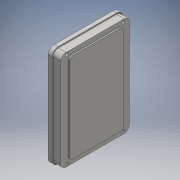
# Autodesk Inventor part: ET6
Saved by Autodesk Inventor 2016 (Build 200138000, 138)
## iProperties
Created: 2016-03-20
Part Number: ET6
Material: Genérico
Document SubType Name: Modeling
Designer: Usuario1
Density: 1 g/cm^3
Appearance: Valor por defecto
Author: Usuario1
Autodesk Inventor part; units mm, degrees
ref_plane "YZ Plane" through (0, 0, 0) normal (1, 0, 0) x (0, 1, 0)
ref_plane "XZ Plane" through (0, 0, 0) normal (0, 1, 0) x (-1, 0, 0)
ref_plane "XY Plane" through (0, 0, 0) normal (0, 0, 1) x (1, 0, 0)
sketch "Boceto1" plane through (0, 0, 0) normal (1, 0, 0) x (0, 1, 0)
  circle A0 centre (0.2799, 0.1054) radius 0.0623
  circle A1 centre (2.483, 0.1054) radius 0.0623
  circle A2 centre (2.483, -3.5918) radius 0.0623
  line L0 (0.3357, -3.3718) -> (0.3357, -0.1146)
  arc A3 (0.3357, -3.3718) -> (0.4557, -3.4918) centre (0.4557, -3.3718) ccw
  line L1 (0.4557, 0.0054) -> (2.3072, 0.0054)
  arc A4 (0.4557, 0.0054) -> (0.3357, -0.1146) centre (0.4557, -0.1146) ccw
  arc A5 (2.4272, -0.1146) -> (2.3072, 0.0054) centre (2.3072, -0.1146) ccw
  line L2 (2.4272, -0.1146) -> (2.4272, -3.3718)
  arc A6 (2.3072, -3.4918) -> (2.4272, -3.3718) centre (2.3072, -3.3718) ccw
  line L3 (2.3072, -3.4918) -> (0.4557, -3.4918)
  line L4 (0, -3.4863) -> (0, 0)
  arc A7 (0.24, 0.24) -> (0, 0) centre (0.24, 0) ccw
  line L5 (0.24, 0.24) -> (2.5229, 0.24)
  arc A8 (2.7629, 0) -> (2.5229, 0.24) centre (2.5229, 0) ccw
  line L6 (2.7629, 0) -> (2.7629, -3.4863)
  arc A9 (2.5229, -3.7263) -> (2.7629, -3.4863) centre (2.5229, -3.4863) ccw
  line L7 (2.5229, -3.7263) -> (0.24, -3.7263)
  arc A10 (0, -3.4863) -> (0.24, -3.7263) centre (0.24, -3.4863) ccw
  line L8 (2.7186, -3.4821) -> (2.7186, -0.0043)
  arc A11 (2.7186, -0.0043) -> (2.5186, 0.1957) centre (2.5186, -0.0043) ccw
  line L9 (2.5186, 0.1957) -> (0.2443, 0.1957)
  arc A12 (0.2443, 0.1957) -> (0.0443, -0.0043) centre (0.2443, -0.0043) ccw
  line L10 (0.0443, -0.0043) -> (0.0443, -3.4821)
  arc A13 (0.0443, -3.4821) -> (0.2443, -3.6821) centre (0.2443, -3.4821) ccw
  line L11 (0.2443, -3.6821) -> (2.5186, -3.6821)
  arc A14 (2.5186, -3.6821) -> (2.7186, -3.4821) centre (2.5186, -3.4821) ccw
  circle A15 centre (0.2799, -3.5918) radius 0.0623
  constraints: 24 end point, 24 point on circle, 16 centre point
extrude "Extrusión1" add sketch "Boceto1" along normal blind 0.15 contours L0 A4 L1 A5 L2 A6 L3 A3 | L4 A7 L5 A8 L6 A9 L7 A10 | A14 L11 A13 L10 A12 L9 A11 L8
sketch "Boceto2" plane through (0.15, 0, 0) normal (1, 0, 0) x (0, 0, -1)
  circle A0 centre (3.5918, 2.483) radius 0.0623
  circle A1 centre (3.5918, 0.2799) radius 0.0623
  circle A2 centre (-0.1054, 0.2799) radius 0.0623
  line L0 (0.1146, 2.4272) -> (3.3718, 2.4272)
  arc A3 (0.1146, 2.4272) -> (-0.0054, 2.3072) centre (0.1146, 2.3072) ccw
  line L1 (3.4918, 2.3072) -> (3.4918, 0.4557)
  arc A4 (3.4918, 2.3072) -> (3.3718, 2.4272) centre (3.3718, 2.3072) ccw
  arc A5 (3.3718, 0.3357) -> (3.4918, 0.4557) centre (3.3718, 0.4557) ccw
  line L2 (3.3718, 0.3357) -> (0.1146, 0.3357)
  arc A6 (-0.0054, 0.4557) -> (0.1146, 0.3357) centre (0.1146, 0.4557) ccw
  line L3 (-0.0054, 0.4557) -> (-0.0054, 2.3072)
  line L4 (0, 2.7629) -> (3.4863, 2.7629)
  arc A7 (3.7263, 2.5229) -> (3.4863, 2.7629) centre (3.4863, 2.5229) ccw
  line L5 (3.7263, 2.5229) -> (3.7263, 0.24)
  arc A8 (3.4863, 0) -> (3.7263, 0.24) centre (3.4863, 0.24) ccw
  line L6 (3.4863, 0) -> (0, 0)
  arc A9 (-0.24, 0.24) -> (0, 0) centre (0, 0.24) ccw
  line L7 (-0.24, 0.24) -> (-0.24, 2.5229)
  arc A10 (0, 2.7629) -> (-0.24, 2.5229) centre (0, 2.5229) ccw
  line L8 (0.0043, 0.0443) -> (3.4821, 0.0443)
  arc A11 (3.4821, 0.0443) -> (3.6821, 0.2443) centre (3.4821, 0.2443) ccw
  line L9 (3.6821, 0.2443) -> (3.6821, 2.5186)
  arc A12 (3.6821, 2.5186) -> (3.4821, 2.7186) centre (3.4821, 2.5186) ccw
  line L10 (3.4821, 2.7186) -> (0.0043, 2.7186)
  arc A13 (0.0043, 2.7186) -> (-0.1957, 2.5186) centre (0.0043, 2.5186) ccw
  line L11 (-0.1957, 2.5186) -> (-0.1957, 0.2443)
  arc A14 (-0.1957, 0.2443) -> (0.0043, 0.0443) centre (0.0043, 0.2443) ccw
  circle A15 centre (-0.1054, 2.483) radius 0.0623
  circle A16 centre (3.5918, 0.2799) radius 0.0623 projected
  circle A17 centre (3.5918, 2.483) radius 0.0623 projected
  circle A18 centre (-0.1054, 2.483) radius 0.0623 projected
  circle A19 centre (-0.1054, 0.2799) radius 0.0623 projected
  line L12 (0, 0) -> (3.4863, 0) projected
  arc A20 (3.4863, 0) -> (3.7263, 0.24) centre (3.4863, 0.24) ccw projected
  line L13 (3.7263, 0.24) -> (3.7263, 2.5229) projected
  arc A21 (3.7263, 2.5229) -> (3.4863, 2.7629) centre (3.4863, 2.5229) ccw projected
  line L14 (3.4863, 2.7629) -> (0, 2.7629) projected
  arc A22 (0, 2.7629) -> (-0.24, 2.5229) centre (0, 2.5229) ccw projected
  line L15 (-0.24, 2.5229) -> (-0.24, 0.24) projected
  arc A23 (-0.24, 0.24) -> (0, 0) centre (0, 0.24) ccw projected
  constraints: 24 end point, 24 point on circle, 16 centre point
extrude "Extrusión2" add sketch "Boceto2" along normal blind 0.3 contours L0 A4 L1 A5 L2 A6 L3 A3 | A14 L11 A13 L10 A12 L9 A11 L8
sketch "Boceto3" plane through (0.45, 0, 0) normal (1, 0, 0) x (0, 0, -1)
  circle A0 centre (-0.1054, 2.483) radius 0.0623 projected
  circle A1 centre (-0.1054, 0.2799) radius 0.0623 projected
  circle A2 centre (3.5918, 0.2799) radius 0.0623 projected
  circle A3 centre (3.5918, 2.483) radius 0.0623 projected
  line L0 (0.0043, 0.0443) -> (3.4821, 0.0443) projected
  arc A4 (3.4821, 0.0443) -> (3.6821, 0.2443) centre (3.4821, 0.2443) ccw projected
  line L1 (3.6821, 0.2443) -> (3.6821, 2.5186) projected
  arc A5 (3.6821, 2.5186) -> (3.4821, 2.7186) centre (3.4821, 2.5186) ccw projected
  line L2 (3.4821, 2.7186) -> (0.0043, 2.7186) projected
  arc A6 (0.0043, 2.7186) -> (-0.1957, 2.5186) centre (0.0043, 2.5186) ccw projected
  line L3 (-0.1957, 2.5186) -> (-0.1957, 0.2443) projected
  arc A7 (-0.1957, 0.2443) -> (0.0043, 0.0443) centre (0.0043, 0.2443) ccw projected
  circle A8 centre (3.5918, 2.483) radius 0.0623
  circle A9 centre (3.5918, 0.2799) radius 0.0623
  circle A10 centre (-0.1054, 0.2799) radius 0.0623
  line L4 (0.1146, 2.4272) -> (3.3718, 2.4272)
  arc A11 (0.1146, 2.4272) -> (-0.0054, 2.3072) centre (0.1146, 2.3072) ccw
  line L5 (3.4918, 2.3072) -> (3.4918, 0.4557)
  arc A12 (3.4918, 2.3072) -> (3.3718, 2.4272) centre (3.3718, 2.3072) ccw
  arc A13 (3.3718, 0.3357) -> (3.4918, 0.4557) centre (3.3718, 0.4557) ccw
  line L6 (3.3718, 0.3357) -> (0.1146, 0.3357)
  arc A14 (-0.0054, 0.4557) -> (0.1146, 0.3357) centre (0.1146, 0.4557) ccw
  line L7 (-0.0054, 0.4557) -> (-0.0054, 2.3072)
  line L8 (0, 2.7629) -> (3.4863, 2.7629)
  arc A15 (3.7263, 2.5229) -> (3.4863, 2.7629) centre (3.4863, 2.5229) ccw
  line L9 (3.7263, 2.5229) -> (3.7263, 0.24)
  arc A16 (3.4863, 0) -> (3.7263, 0.24) centre (3.4863, 0.24) ccw
  line L10 (3.4863, 0) -> (0, 0)
  arc A17 (-0.24, 0.24) -> (0, 0) centre (0, 0.24) ccw
  line L11 (-0.24, 0.24) -> (-0.24, 2.5229)
  arc A18 (0, 2.7629) -> (-0.24, 2.5229) centre (0, 2.5229) ccw
  line L12 (0.0043, 0.0443) -> (3.4821, 0.0443)
  arc A19 (3.4821, 0.0443) -> (3.6821, 0.2443) centre (3.4821, 0.2443) ccw
  line L13 (3.6821, 0.2443) -> (3.6821, 2.5186)
  arc A20 (3.6821, 2.5186) -> (3.4821, 2.7186) centre (3.4821, 2.5186) ccw
  line L14 (3.4821, 2.7186) -> (0.0043, 2.7186)
  arc A21 (0.0043, 2.7186) -> (-0.1957, 2.5186) centre (0.0043, 2.5186) ccw
  line L15 (-0.1957, 2.5186) -> (-0.1957, 0.2443)
  arc A22 (-0.1957, 0.2443) -> (0.0043, 0.0443) centre (0.0043, 0.2443) ccw
  circle A23 centre (-0.1054, 2.483) radius 0.0623
  point P0 (0, 0)
  constraints: 24 end point, 24 point on circle, 16 centre point
extrude "Extrusión3" add sketch "Boceto3" along normal blind 0.05 contours L4 A12 L5 A13 L6 A14 L7 A11
